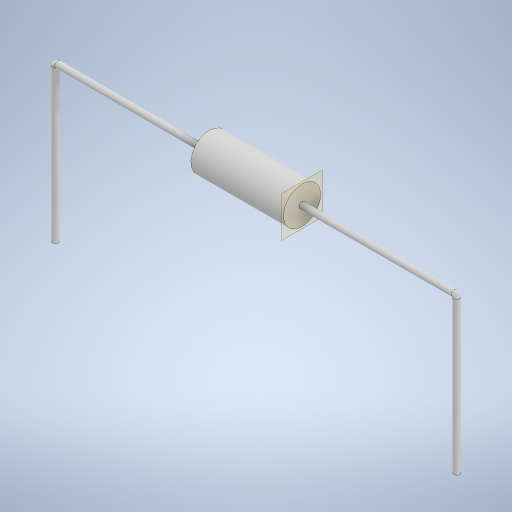
# Autodesk Inventor part: КС147А
Saved by Autodesk Inventor 2024 (Build 280153000, 153)
## iProperties
Created: 2023-12-04
Part Number: КС147А
Material: Типовые
Document SubType Name: Modeling
Designer: SaNe4Ka
Density: 1 g/cm^3
Appearance: По умолчанию
Author: SaNe4Ka
Autodesk Inventor part; units mm, degrees
ref_plane "YZ Plane" through (0, 0, 0) normal (1, 0, 0) x (0, 1, 0)
ref_plane "XZ Plane" through (0, 0, 0) normal (0, 1, 0) x (-1, 0, 0)
ref_plane "XY Plane" through (0, 0, 0) normal (0, 0, 1) x (1, 0, 0)
sketch "Эскиз1" plane through (0, 0, 0) normal (0, 0, 1) x (1, 0, 0)
  line L0 (-3.7707, 0) -> (-3.7707, 1.5)
  line L1 (-3.7707, 1.5) -> (3.7293, 1.5)
  line L2 (3.7293, 1.5) -> (3.7293, 0)
  line L3 (3.7293, 0) -> (-3.7707, 0)
  point P0 (0, 0)
  dimension "d0" = 1.5
  dimension "d1" = 7.5
  constraints: 8 end point, 3 perpendicular, 1 vertical
  measures "d0" distance of L0.start L0.end
  measures "d1" distance of L0.end L1.end
revolve "Вращение1" add sketch "Эскиз1" angle 360 about axis through (3.7293, 0, 0) along (-1, 0, 0)
sketch "Эскиз4" plane through (0, 0, 0) normal (0, 0, 1) x (1, 0, 0)
  line L0 (3.7293, 1.5) -> (3.7293, -1.5) projected
  line L1 (3.7293, 0) -> (16.0293, 0)
  line L2 (16.2293, -0.2) -> (16.2293, -12.5)
  arc A0 (16.2293, -0.2) -> (16.0293, 0) centre (16.0293, -0.2) ccw
  point P0 (0, 0)
  point P1 (16.2293, 0)
  dimension "d3" = 12.5
  dimension "d4" = 12.5
  dimension "d5" = 0.2
  constraints: 4 end point, 2 point on circle, 2 point on line, 2 tangent, 1 centre point, 1 horizontal, 1 midpoint, 1 perpendicular
  measures "d3" distance of L1.start point (16.229, 0)
  measures "d4" distance of point (16.229, 0) L2.end
  measures "d5" radius of A0
ref_plane "РабПлоскость1" through (3.7293, 0, 0) normal (1, 0, 0) x (0, 0, -1)
sketch "Эскиз5" plane through (3.7293, 0, 0) normal (1, 0, 0) x (0, 0, -1)
  circle A0 centre (0, 0) radius 0.25
  dimension "d7" = 0.5
  constraints: 1 centre point, 1 coincident
  measures "d7" diameter of A0
sweep "Сдвиг1" add profiles "Эскиз5" path "Эскиз4" path curves L1 A0 L2
mirror "Зеркальное отражение1" about plane through (0, 0, 0) normal (1, 0, 0) of "Сдвиг1"
